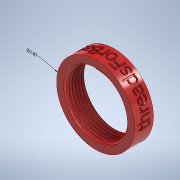
# Autodesk Inventor part: threadsForBaseV04
Saved by Autodesk Inventor 2021.1 (Build 251245010, 245A)
## iProperties
Created: 2020-08-18
Part Number: threadsForBaseV04
Material: PET Plastic
Document SubType Name: Modeling
Designer: robst
Density: 1.541 g/cm^3
Appearance: Red
Author: robst
Autodesk Inventor part; units mm, degrees
ref_plane "YZ Plane" through (0, 0, 0) normal (1, 0, 0) x (0, 1, 0)
ref_plane "XY Plane" through (0, 0, 0) normal (0, 0, 1) x (1, 0, 0)
sketch "Sketch3" plane through (0, 0, 0) normal (0, 0, 1) x (1, 0, 0)
  circle A0 centre (0, 0) radius 8.0645
  circle A1 centre (0, 0) radius 26.3436
  dimension "d8" = 16.129
  dimension "d9" = 52.6872
  constraints: 2 centre point, 2 coincident
  measures "d8" diameter of A0
  measures "d9" diameter of A1
extrude "Extrusion3" add sketch "Sketch3" along normal blind 44.45
sketch "Sketch4" plane through (0, 0, 44.45) normal (0, 0, 1) x (1, 0, 0)
  circle A0 centre (0, 0) radius 21.5811
  dimension "d12" = 43.1622
  constraints: 1 centre point, 1 coincident
  measures "d12" diameter of A0
extrude "Extrusion4" cut sketch "Sketch4" against normal blind 31.75
sketch "Sketch5" plane through (0, 0, 0) normal (1, 0, 0) x (0, 1, 0)
  line L0 (21.5811, 44.45) -> (21.5811, 12.7) projected
  line L1 (26.3436, 44.45) -> (-26.3436, 44.45) projected
  line L2 (21.5811, 44.45) -> (21.5811, 44.45)
  line L3 (21.5811, 44.45) -> (20.4572, 43.8011)
  line L4 (20.4572, 43.6031) -> (21.5811, 42.9542)
  arc A0 (20.4572, 43.8011) -> (20.4572, 43.6031) centre (20.5143, 43.7021) ccw
  line L5 (0, -8.89) -> (0, 53.34) construction
  line L6 (21.5811, 42.9542) -> (21.5811, 44.45)
  point P0 (0, 0)
  dimension "d15" = 60
  dimension "d17" = 0.1143
  dimension "d18" = 20.4
  dimension "d27" = 0
  constraints: 8 end point, 2 point on circle, 2 tangent, 1 centre point, 1 collinear, 1 equal length, 1 point on line, 1 vertical
  measures "d15" angle of L4 L3
  measures "d17" radius of A0
  measures "d18" distance edge to line of A0 L5
  measures "d27" distance of L2.end L0.start
coil "Coil2" sketch "Sketch5" operation add axis through (0, 0, -10) along (0, 0, -1) pitch 2.1167 turns 15 hand right
ref_plane "Work Plane3" through (0, 0, 31.75) normal (0, 0, 1) x (1, 0, 0)
sketch "Sketch12" plane through (0, 0, 31.75) normal (0, 0, 1) x (1, 0, 0)
  circle A0 centre (0, 0) radius 26.9875
  constraints: 1 centre point, 1 coincident
extrude "Extrusion7" cut sketch "Sketch12" against normal through all
ref_plane "Work Plane5" through (0, 26.3436, 0) normal (0, 1, 0) x (-1, 0, 0)
sketch "Sketch15" plane through (0, 26.3436, 0) normal (0, 1, 0) x (-1, 0, 0)
  line L0 (-26.3436, 31.75) -> (-26.3436, 44.45) projected
  line L1 (26.3436, 31.75) -> (26.3436, 44.45) projected
  line L2 (-26.3436, 38.1) -> (26.3436, 38.1) construction
  spline S0 degree 2 poles (-43.7594, 34.1788) (-44.5437, 34.1788) (-45.4267, 35.0742) (-45.4267, 36.0437) knots 0 0 0 1 2 2 2
  line L3 (-45.4267, 36.0437) -> (-45.4267, 39.2115)
  line L4 (-45.4267, 39.2115) -> (-46.0751, 39.2115)
  line L5 (-46.0751, 39.2115) -> (-46.0751, 40.0081)
  line L6 (-46.0751, 40.0081) -> (-45.4267, 40.0081)
  line L7 (-45.4267, 40.0081) -> (-45.4267, 41.6506)
  line L8 (-45.4267, 41.6506) -> (-44.4634, 41.6506)
  line L9 (-44.4634, 41.6506) -> (-44.4634, 40.0081)
  line L10 (-44.4634, 40.0081) -> (-42.6911, 40.0081)
  line L11 (-42.6911, 40.0081) -> (-42.6911, 39.2115)
  line L12 (-42.6911, 39.2115) -> (-44.4634, 39.2115)
  line L13 (-44.4634, 39.2115) -> (-44.4634, 36.4883)
  spline S1 degree 2 poles (-44.4634, 36.4883) (-44.4634, 36.0561) (-44.4325, 35.5806) (-44.3275, 35.3768) knots 0 0 0 1 2 2 2
  spline S2 degree 2 poles (-44.3275, 35.3768) (-44.2411, 35.1977) (-43.8521, 35.0187) (-43.5186, 35.0187) knots 0 0 0 1 2 2 2
  spline S3 degree 2 poles (-43.5186, 35.0187) (-43.2839, 35.0187) (-42.8455, 35.1607) (-42.7467, 35.2039) knots 0 0 0 1 2 2 2
  line L14 (-42.7467, 35.2039) -> (-42.6911, 35.2039)
  line L15 (-42.6911, 35.2039) -> (-42.6911, 34.3394)
  spline S4 degree 2 poles (-42.6911, 34.3394) (-42.9628, 34.2653) (-43.5186, 34.1788) (-43.7594, 34.1788) knots 0 0 0 1 2 2 2
  line L16 (-37.4918, 34.29) -> (-38.4551, 34.29)
  line L17 (-38.4551, 34.29) -> (-38.4551, 37.5504)
  spline S5 degree 2 poles (-38.4551, 37.5504) (-38.4551, 37.9456) (-38.5292, 38.6249) (-38.6403, 38.8287) knots 0 0 0 1 2 2 2
  spline S6 degree 2 poles (-38.6403, 38.8287) (-38.7576, 39.0448) (-39.1775, 39.2547) (-39.5357, 39.2547) knots 0 0 0 1 2 2 2
  spline S7 degree 2 poles (-39.5357, 39.2547) (-39.8939, 39.2547) (-40.6534, 38.8719) (-41.0177, 38.5631) knots 0 0 0 1 2 2 2
  line L18 (-41.0177, 38.5631) -> (-41.0177, 34.29)
  line L19 (-41.0177, 34.29) -> (-41.981, 34.29)
  line L20 (-41.981, 34.29) -> (-41.981, 42.2496)
  line L21 (-41.981, 42.2496) -> (-41.0177, 42.2496)
  line L22 (-41.0177, 42.2496) -> (-41.0177, 39.3721)
  spline S8 degree 2 poles (-41.0177, 39.3721) (-40.5855, 39.7611) (-39.7518, 40.1686) (-39.2825, 40.1686) knots 0 0 0 1 2 2 2
  spline S9 degree 2 poles (-39.2825, 40.1686) (-38.4427, 40.1686) (-37.4918, 39.0571) (-37.4918, 38.0012) knots 0 0 0 1 2 2 2
  line L23 (-37.4918, 38.0012) -> (-37.4918, 34.29)
  line L24 (-33.1075, 38.9769) -> (-33.1569, 38.9769)
  spline S10 degree 2 poles (-33.1569, 38.9769) (-33.268, 39.0077) (-33.5089, 39.0201) (-33.6756, 39.0201) knots 0 0 0 1 2 2 2
  spline S11 degree 2 poles (-33.6756, 39.0201) (-34.0646, 39.0201) (-34.8303, 38.6805) (-35.1761, 38.347) knots 0 0 0 1 2 2 2
  line L25 (-35.1761, 38.347) -> (-35.1761, 34.29)
  line L26 (-35.1761, 34.29) -> (-36.1394, 34.29)
  line L27 (-36.1394, 34.29) -> (-36.1394, 40.0081)
  line L28 (-36.1394, 40.0081) -> (-35.1761, 40.0081)
  line L29 (-35.1761, 40.0081) -> (-35.1761, 39.1559)
  spline S12 degree 2 poles (-35.1761, 39.1559) (-34.6512, 39.6252) (-33.867, 40.0081) (-33.4965, 40.0081) knots 0 0 0 1 2 2 2
  spline S13 degree 2 poles (-33.4965, 40.0081) (-33.3483, 40.0081) (-33.2001, 39.9957) (-33.1075, 39.9772) knots 0 0 0 1 2 2 2
  line L30 (-33.1075, 39.9772) -> (-33.1075, 38.9769)
  spline S14 degree 2 poles (-29.8779, 34.1603) (-31.2488, 34.1603) (-32.7555, 35.6979) (-32.7555, 37.1182) knots 0 0 0 1 2 2 2
  spline S15 degree 2 poles (-32.7555, 37.1182) (-32.7555, 38.5137) (-31.292, 40.1686) (-30.1126, 40.1686) knots 0 0 0 1 2 2 2
  spline S16 degree 2 poles (-30.1126, 40.1686) (-29.5815, 40.1686) (-28.7603, 39.8599) (-28.4577, 39.5326) knots 0 0 0 1 2 2 2
  spline S17 degree 2 poles (-28.4577, 39.5326) (-28.1489, 39.2053) (-27.8216, 38.2606) (-27.8216, 37.5751) knots 0 0 0 1 2 2 2
  line L31 (-27.8216, 37.5751) -> (-27.8216, 37.0502)
  line L32 (-27.8216, 37.0502) -> (-31.7798, 37.0502)
  spline S18 degree 2 poles (-31.7798, 37.0502) (-31.7798, 36.0561) (-30.7795, 35.0001) (-29.8903, 35.0001) knots 0 0 0 1 2 2 2
  spline S19 degree 2 poles (-29.8903, 35.0001) (-29.5754, 35.0001) (-28.964, 35.1422) (-28.717, 35.2533) knots 0 0 0 1 2 2 2
  spline S20 degree 2 poles (-28.717, 35.2533) (-28.4577, 35.3768) (-28.0995, 35.5929) (-27.9822, 35.6917) knots 0 0 0 1 2 2 2
  line L33 (-27.9822, 35.6917) -> (-27.9266, 35.6917)
  line L34 (-27.9266, 35.6917) -> (-27.9266, 34.642)
  spline S21 degree 2 poles (-27.9266, 34.642) (-28.0933, 34.5741) (-28.5997, 34.3765) (-28.7973, 34.3209) knots 0 0 0 1 2 2 2
  spline S22 degree 2 poles (-28.7973, 34.3209) (-29.0752, 34.2406) (-29.5321, 34.1603) (-29.8779, 34.1603) knots 0 0 0 1 2 2 2
  spline S23 degree 2 poles (-28.7603, 37.7851) (-28.7726, 38.1741) (-28.9332, 38.7422) (-29.0875, 38.9336) knots 0 0 0 1 2 2 2
  spline S24 degree 2 poles (-29.0875, 38.9336) (-29.2543, 39.1498) (-29.7791, 39.3782) (-30.1682, 39.3782) knots 0 0 0 1 2 2 2
  spline S25 degree 2 poles (-30.1682, 39.3782) (-30.551, 39.3782) (-31.0882, 39.1498) (-31.3105, 38.9275) knots 0 0 0 1 2 2 2
  spline S26 degree 2 poles (-31.3105, 38.9275) (-31.5267, 38.699) (-31.749, 38.1494) (-31.7798, 37.7851) knots 0 0 0 1 2 2 2
  line L35 (-31.7798, 37.7851) -> (-28.7603, 37.7851)
  spline S27 degree 2 poles (-23.6597, 34.8952) (-23.777, 34.8087) (-24.1722, 34.5) (-24.3574, 34.4073) knots 0 0 0 1 2 2 2
  spline S28 degree 2 poles (-24.3574, 34.4073) (-24.6106, 34.2715) (-25.0861, 34.1294) (-25.5184, 34.1294) knots 0 0 0 1 2 2 2
  spline S29 degree 2 poles (-25.5184, 34.1294) (-25.8703, 34.1294) (-26.5064, 34.395) (-26.7472, 34.6358) knots 0 0 0 1 2 2 2
  spline S30 degree 2 poles (-26.7472, 34.6358) (-26.9757, 34.8705) (-27.2535, 35.5621) (-27.2535, 35.9449) knots 0 0 0 1 2 2 2
  spline S31 degree 2 poles (-27.2535, 35.9449) (-27.2535, 36.5377) (-26.7534, 37.3775) (-26.21, 37.6183) knots 0 0 0 1 2 2 2
  spline S32 degree 2 poles (-26.21, 37.6183) (-25.7283, 37.8406) (-24.4192, 38.0074) (-23.6597, 38.0506) knots 0 0 0 1 2 2 2
  line L36 (-23.6597, 38.0506) -> (-23.6597, 38.2359)
  spline S33 degree 2 poles (-23.6597, 38.2359) (-23.6597, 38.5693) (-23.8634, 38.983) (-24.0487, 39.1004) knots 0 0 0 1 2 2 2
  spline S34 degree 2 poles (-24.0487, 39.1004) (-24.2339, 39.2177) (-24.765, 39.2918) (-25.0491, 39.2918) knots 0 0 0 1 2 2 2
  spline S35 degree 2 poles (-25.0491, 39.2918) (-25.3825, 39.2918) (-26.2841, 39.0942) (-26.7348, 38.9028) knots 0 0 0 1 2 2 2
  line L37 (-26.7348, 38.9028) -> (-26.7904, 38.9028)
  line L38 (-26.7904, 38.9028) -> (-26.7904, 39.8846)
  spline S36 degree 2 poles (-26.7904, 39.8846) (-26.5249, 39.9587) (-25.5307, 40.1439) (-25.0429, 40.1439) knots 0 0 0 1 2 2 2
  spline S37 degree 2 poles (-25.0429, 40.1439) (-24.4501, 40.1439) (-23.6411, 39.9587) (-23.32, 39.7179) knots 0 0 0 1 2 2 2
  spline S38 degree 2 poles (-23.32, 39.7179) (-23.0051, 39.4832) (-22.6964, 38.736) (-22.6964, 38.1988) knots 0 0 0 1 2 2 2
  line L39 (-22.6964, 38.1988) -> (-22.6964, 34.29)
  line L40 (-22.6964, 34.29) -> (-23.6597, 34.29)
  line L41 (-23.6597, 34.29) -> (-23.6597, 34.8952)
  line L42 (-23.6597, 35.6979) -> (-23.6597, 37.2849)
  spline S39 degree 2 poles (-23.6597, 37.2849) (-24.0055, 37.254) (-25.0491, 37.149) (-25.3763, 37.0502) knots 0 0 0 1 2 2 2
  spline S40 degree 2 poles (-25.3763, 37.0502) (-25.7592, 36.9329) (-26.2594, 36.4451) (-26.2594, 36.0128) knots 0 0 0 1 2 2 2
  spline S41 degree 2 poles (-26.2594, 36.0128) (-26.2594, 35.5188) (-25.7036, 35.0187) (-25.1726, 35.0187) knots 0 0 0 1 2 2 2
  spline S42 degree 2 poles (-25.1726, 35.0187) (-24.7218, 35.0187) (-23.9808, 35.4077) (-23.6597, 35.6979) knots 0 0 0 1 2 2 2
  line L43 (-16.9474, 34.29) -> (-17.9107, 34.29)
  line L44 (-17.9107, 34.29) -> (-17.9107, 34.8705)
  spline S43 degree 2 poles (-17.9107, 34.8705) (-18.133, 34.6852) (-18.4603, 34.4382) (-18.6826, 34.3332) knots 0 0 0 1 2 2 2
  spline S44 degree 2 poles (-18.6826, 34.3332) (-18.8864, 34.2344) (-19.3248, 34.1294) (-19.615, 34.1294) knots 0 0 0 1 2 2 2
  spline S45 degree 2 poles (-19.615, 34.1294) (-20.0843, 34.1294) (-20.8747, 34.5185) (-21.1526, 34.8952) knots 0 0 0 1 2 2 2
  spline S46 degree 2 poles (-21.1526, 34.8952) (-21.4305, 35.2718) (-21.7392, 36.3833) (-21.7392, 37.1058) knots 0 0 0 1 2 2 2
  spline S47 degree 2 poles (-21.7392, 37.1058) (-21.7392, 37.8592) (-21.3502, 38.9583) (-21.0106, 39.3721) knots 0 0 0 1 2 2 2
  spline S48 degree 2 poles (-21.0106, 39.3721) (-20.6957, 39.7426) (-19.8126, 40.1686) (-19.3248, 40.1686) knots 0 0 0 1 2 2 2
  spline S49 degree 2 poles (-19.3248, 40.1686) (-18.8987, 40.1686) (-18.2627, 39.9772) (-17.9107, 39.7796) knots 0 0 0 1 2 2 2
  line L45 (-17.9107, 39.7796) -> (-17.9107, 42.2496)
  line L46 (-17.9107, 42.2496) -> (-16.9474, 42.2496)
  line L47 (-16.9474, 42.2496) -> (-16.9474, 34.29)
  line L48 (-17.9107, 35.6794) -> (-17.9107, 38.983)
  spline S50 degree 2 poles (-17.9107, 38.983) (-18.2689, 39.1559) (-18.837, 39.2856) (-19.1642, 39.2856) knots 0 0 0 1 2 2 2
  spline S51 degree 2 poles (-19.1642, 39.2856) (-19.9052, 39.2856) (-20.7451, 38.1741) (-20.7451, 37.1243) knots 0 0 0 1 2 2 2
  spline S52 degree 2 poles (-20.7451, 37.1243) (-20.7451, 36.1116) (-20.1028, 35.0434) (-19.3927, 35.0434) knots 0 0 0 1 2 2 2
  spline S53 degree 2 poles (-19.3927, 35.0434) (-19.016, 35.0434) (-18.2503, 35.3892) (-17.9107, 35.6794) knots 0 0 0 1 2 2 2
  spline S54 degree 2 poles (-14.0081, 34.1541) (-14.5824, 34.1541) (-15.5765, 34.4629) (-15.9038, 34.6358) knots 0 0 0 1 2 2 2
  line L49 (-15.9038, 34.6358) -> (-15.9038, 35.7164)
  line L50 (-15.9038, 35.7164) -> (-15.8544, 35.7164)
  spline S55 degree 2 poles (-15.8544, 35.7164) (-15.7309, 35.6176) (-15.3975, 35.383) (-15.1196, 35.2533) knots 0 0 0 1 2 2 2
  spline S56 degree 2 poles (-15.1196, 35.2533) (-14.8788, 35.136) (-14.286, 34.9631) (-13.971, 34.9631) knots 0 0 0 1 2 2 2
  spline S57 degree 2 poles (-13.971, 34.9631) (-13.7426, 34.9631) (-13.2177, 35.0681) (-13.0942, 35.1545) knots 0 0 0 1 2 2 2
  spline S58 degree 2 poles (-13.0942, 35.1545) (-12.9151, 35.2718) (-12.7545, 35.5374) (-12.7545, 35.8091) knots 0 0 0 1 2 2 2
  spline S59 degree 2 poles (-12.7545, 35.8091) (-12.7545, 36.1487) (-13.1251, 36.5007) (-13.6005, 36.618) knots 0 0 0 1 2 2 2
  spline S60 degree 2 poles (-13.6005, 36.618) (-13.7858, 36.6612) (-14.3786, 36.7847) (-14.6318, 36.8526) knots 0 0 0 1 2 2 2
  spline S61 degree 2 poles (-14.6318, 36.8526) (-15.2863, 37.0441) (-15.8791, 37.8345) (-15.8791, 38.3964) knots 0 0 0 1 2 2 2
  spline S62 degree 2 poles (-15.8791, 38.3964) (-15.8791, 39.1745) (-14.712, 40.1439) (-13.7487, 40.1439) knots 0 0 0 1 2 2 2
  spline S63 degree 2 poles (-13.7487, 40.1439) (-13.2733, 40.1439) (-12.3099, 39.9093) (-11.9827, 39.7302) knots 0 0 0 1 2 2 2
  line L51 (-11.9827, 39.7302) -> (-11.9827, 38.699)
  line L52 (-11.9827, 38.699) -> (-12.0321, 38.699)
  spline S64 degree 2 poles (-12.0321, 38.699) (-12.4026, 38.9954) (-13.3041, 39.335) (-13.7673, 39.335) knots 0 0 0 1 2 2 2
  spline S65 degree 2 poles (-13.7673, 39.335) (-14.2427, 39.335) (-14.8973, 38.9336) (-14.8973, 38.5323) knots 0 0 0 1 2 2 2
  spline S66 degree 2 poles (-14.8973, 38.5323) (-14.8973, 38.1679) (-14.5083, 37.8159) (-14.076, 37.7048) knots 0 0 0 1 2 2 2
  spline S67 degree 2 poles (-14.076, 37.7048) (-13.8661, 37.6492) (-13.335, 37.5381) (-13.0448, 37.4701) knots 0 0 0 1 2 2 2
  spline S68 degree 2 poles (-13.0448, 37.4701) (-12.4149, 37.3096) (-11.7727, 36.5748) (-11.7727, 35.9387) knots 0 0 0 1 2 2 2
  spline S69 degree 2 poles (-11.7727, 35.9387) (-11.7727, 35.5682) (-12.0629, 34.9137) (-12.347, 34.6729) knots 0 0 0 1 2 2 2
  spline S70 degree 2 poles (-12.347, 34.6729) (-12.6496, 34.4197) (-13.4215, 34.1541) (-14.0081, 34.1541) knots 0 0 0 1 2 2 2
  line L53 (-6.2461, 41.0084) -> (-9.7905, 41.0084)
  line L54 (-9.7905, 41.0084) -> (-9.7905, 38.8595)
  line L55 (-9.7905, 38.8595) -> (-6.3943, 38.8595)
  line L56 (-6.3943, 38.8595) -> (-6.3943, 37.958)
  line L57 (-6.3943, 37.958) -> (-9.7905, 37.958)
  line L58 (-9.7905, 37.958) -> (-9.7905, 34.29)
  line L59 (-9.7905, 34.29) -> (-10.8032, 34.29)
  line L60 (-10.8032, 34.29) -> (-10.8032, 41.91)
  line L61 (-10.8032, 41.91) -> (-6.2461, 41.91)
  line L62 (-6.2461, 41.91) -> (-6.2461, 41.0084)
  spline S71 degree 2 poles (-0.7132, 37.149) (-0.7132, 35.7041) (-2.1026, 34.1294) (-3.2635, 34.1294) knots 0 0 0 1 2 2 2
  spline S72 degree 2 poles (-3.2635, 34.1294) (-4.4553, 34.1294) (-5.82, 35.7535) (-5.82, 37.149) knots 0 0 0 1 2 2 2
  spline S73 degree 2 poles (-5.82, 37.149) (-5.82, 38.5817) (-4.4121, 40.1686) (-3.2635, 40.1686) knots 0 0 0 1 2 2 2
  spline S74 degree 2 poles (-3.2635, 40.1686) (-2.1026, 40.1686) (-0.7132, 38.5878) (-0.7132, 37.149) knots 0 0 0 1 2 2 2
  spline S75 degree 2 poles (-1.7074, 37.149) (-1.7074, 38.2606) (-2.5163, 39.3412) (-3.2635, 39.3412) knots 0 0 0 1 2 2 2
  spline S76 degree 2 poles (-3.2635, 39.3412) (-4.0107, 39.3412) (-4.8258, 38.2606) (-4.8258, 37.149) knots 0 0 0 1 2 2 2
  spline S77 degree 2 poles (-4.8258, 37.149) (-4.8258, 36.0684) (-4.0107, 34.9569) (-3.2635, 34.9569) knots 0 0 0 1 2 2 2
  spline S78 degree 2 poles (-3.2635, 34.9569) (-2.5225, 34.9569) (-1.7074, 36.0499) (-1.7074, 37.149) knots 0 0 0 1 2 2 2
  line L63 (3.3067, 38.9769) -> (3.2573, 38.9769)
  spline S79 degree 2 poles (3.2573, 38.9769) (3.1462, 39.0077) (2.9054, 39.0201) (2.7386, 39.0201) knots 0 0 0 1 2 2 2
  spline S80 degree 2 poles (2.7386, 39.0201) (2.3496, 39.0201) (1.5839, 38.6805) (1.2381, 38.347) knots 0 0 0 1 2 2 2
  line L64 (1.2381, 38.347) -> (1.2381, 34.29)
  line L65 (1.2381, 34.29) -> (0.2748, 34.29)
  line L66 (0.2748, 34.29) -> (0.2748, 40.0081)
  line L67 (0.2748, 40.0081) -> (1.2381, 40.0081)
  line L68 (1.2381, 40.0081) -> (1.2381, 39.1559)
  spline S81 degree 2 poles (1.2381, 39.1559) (1.763, 39.6252) (2.5472, 40.0081) (2.9177, 40.0081) knots 0 0 0 1 2 2 2
  spline S82 degree 2 poles (2.9177, 40.0081) (3.0659, 40.0081) (3.2141, 39.9957) (3.3067, 39.9772) knots 0 0 0 1 2 2 2
  line L69 (3.3067, 39.9772) -> (3.3067, 38.9769)
  spline S83 degree 2 poles (9.2965, 36.6303) (9.2965, 36.0622) (8.8643, 35.1916) (8.5061, 34.9075) knots 0 0 0 1 2 2 2
  spline S84 degree 2 poles (8.5061, 34.9075) (8.0739, 34.5741) (7.092, 34.29) (6.314, 34.29) knots 0 0 0 1 2 2 2
  line L70 (6.314, 34.29) -> (4.128, 34.29)
  line L71 (4.128, 34.29) -> (4.128, 41.91)
  line L72 (4.128, 41.91) -> (6.1473, 41.91)
  spline S85 degree 2 poles (6.1473, 41.91) (6.9624, 41.91) (7.7775, 41.805) (8.148, 41.6012) knots 0 0 0 1 2 2 2
  spline S86 degree 2 poles (8.148, 41.6012) (8.5617, 41.3851) (8.9384, 40.675) (8.9384, 40.1933) knots 0 0 0 1 2 2 2
  spline S87 degree 2 poles (8.9384, 40.1933) (8.9384, 39.6561) (8.3703, 38.804) (7.8701, 38.5631) knots 0 0 0 1 2 2 2
  line L73 (7.8701, 38.5631) -> (7.8701, 38.5261)
  spline S88 degree 2 poles (7.8701, 38.5261) (8.5493, 38.3408) (9.2965, 37.359) (9.2965, 36.6303) knots 0 0 0 1 2 2 2
  spline S89 degree 2 poles (8.2406, 36.5871) (8.2406, 37.0194) (7.9936, 37.5751) (7.6231, 37.7727) knots 0 0 0 1 2 2 2
  spline S90 degree 2 poles (7.6231, 37.7727) (7.3823, 37.8962) (6.8142, 37.9703) (6.2893, 37.9703) knots 0 0 0 1 2 2 2
  line L74 (6.2893, 37.9703) -> (5.1407, 37.9703)
  line L75 (5.1407, 37.9703) -> (5.1407, 35.1545)
  line L76 (5.1407, 35.1545) -> (5.962, 35.1545)
  spline S91 degree 2 poles (5.962, 35.1545) (6.6289, 35.1545) (7.3946, 35.278) (7.691, 35.4756) knots 0 0 0 1 2 2 2
  spline S92 degree 2 poles (7.691, 35.4756) (7.9751, 35.6794) (8.2406, 36.1857) (8.2406, 36.5871) knots 0 0 0 1 2 2 2
  spline S93 degree 2 poles (7.8824, 40.0513) (7.8824, 40.323) (7.6972, 40.7306) (7.4934, 40.8479) knots 0 0 0 1 2 2 2
  spline S94 degree 2 poles (7.4934, 40.8479) (7.2464, 40.9837) (6.6474, 41.0455) (6.1102, 41.0455) knots 0 0 0 1 2 2 2
  line L77 (6.1102, 41.0455) -> (5.1407, 41.0455)
  line L78 (5.1407, 41.0455) -> (5.1407, 38.8163)
  line L79 (5.1407, 38.8163) -> (6.2893, 38.8163)
  spline S95 degree 2 poles (6.2893, 38.8163) (6.7648, 38.8163) (7.2155, 38.9151) (7.4564, 39.0695) knots 0 0 0 1 2 2 2
  spline S96 degree 2 poles (7.4564, 39.0695) (7.691, 39.2177) (7.8824, 39.6932) (7.8824, 40.0513) knots 0 0 0 1 2 2 2
  spline S97 degree 2 poles (13.4153, 34.8952) (13.2979, 34.8087) (12.9027, 34.5) (12.7175, 34.4073) knots 0 0 0 1 2 2 2
  spline S98 degree 2 poles (12.7175, 34.4073) (12.4643, 34.2715) (11.9888, 34.1294) (11.5566, 34.1294) knots 0 0 0 1 2 2 2
  spline S99 degree 2 poles (11.5566, 34.1294) (11.2046, 34.1294) (10.5686, 34.395) (10.3278, 34.6358) knots 0 0 0 1 2 2 2
  spline S100 degree 2 poles (10.3278, 34.6358) (10.0993, 34.8705) (9.8214, 35.5621) (9.8214, 35.9449) knots 0 0 0 1 2 2 2
  spline S101 degree 2 poles (9.8214, 35.9449) (9.8214, 36.5377) (10.3216, 37.3775) (10.865, 37.6183) knots 0 0 0 1 2 2 2
  spline S102 degree 2 poles (10.865, 37.6183) (11.3466, 37.8406) (12.6557, 38.0074) (13.4153, 38.0506) knots 0 0 0 1 2 2 2
  line L80 (13.4153, 38.0506) -> (13.4153, 38.2359)
  spline S103 degree 2 poles (13.4153, 38.2359) (13.4153, 38.5693) (13.2115, 38.983) (13.0262, 39.1004) knots 0 0 0 1 2 2 2
  spline S104 degree 2 poles (13.0262, 39.1004) (12.841, 39.2177) (12.3099, 39.2918) (12.0259, 39.2918) knots 0 0 0 1 2 2 2
  spline S105 degree 2 poles (12.0259, 39.2918) (11.6924, 39.2918) (10.7909, 39.0942) (10.3401, 38.9028) knots 0 0 0 1 2 2 2
  line L81 (10.3401, 38.9028) -> (10.2845, 38.9028)
  line L82 (10.2845, 38.9028) -> (10.2845, 39.8846)
  spline S106 degree 2 poles (10.2845, 39.8846) (10.5501, 39.9587) (11.5442, 40.1439) (12.0321, 40.1439) knots 0 0 0 1 2 2 2
  spline S107 degree 2 poles (12.0321, 40.1439) (12.6249, 40.1439) (13.4338, 39.9587) (13.7549, 39.7179) knots 0 0 0 1 2 2 2
  spline S108 degree 2 poles (13.7549, 39.7179) (14.0698, 39.4832) (14.3786, 38.736) (14.3786, 38.1988) knots 0 0 0 1 2 2 2
  line L83 (14.3786, 38.1988) -> (14.3786, 34.29)
  line L84 (14.3786, 34.29) -> (13.4153, 34.29)
  line L85 (13.4153, 34.29) -> (13.4153, 34.8952)
  line L86 (13.4153, 35.6979) -> (13.4153, 37.2849)
  spline S109 degree 2 poles (13.4153, 37.2849) (13.0695, 37.254) (12.0259, 37.149) (11.6986, 37.0502) knots 0 0 0 1 2 2 2
  spline S110 degree 2 poles (11.6986, 37.0502) (11.3158, 36.9329) (10.8156, 36.4451) (10.8156, 36.0128) knots 0 0 0 1 2 2 2
  spline S111 degree 2 poles (10.8156, 36.0128) (10.8156, 35.5188) (11.3713, 35.0187) (11.9024, 35.0187) knots 0 0 0 1 2 2 2
  spline S112 degree 2 poles (11.9024, 35.0187) (12.3532, 35.0187) (13.0942, 35.4077) (13.4153, 35.6979) knots 0 0 0 1 2 2 2
  spline S113 degree 2 poles (17.2747, 34.1541) (16.7004, 34.1541) (15.7062, 34.4629) (15.3789, 34.6358) knots 0 0 0 1 2 2 2
  line L87 (15.3789, 34.6358) -> (15.3789, 35.7164)
  line L88 (15.3789, 35.7164) -> (15.4283, 35.7164)
  spline S114 degree 2 poles (15.4283, 35.7164) (15.5518, 35.6176) (15.8853, 35.383) (16.1632, 35.2533) knots 0 0 0 1 2 2 2
  spline S115 degree 2 poles (16.1632, 35.2533) (16.404, 35.136) (16.9968, 34.9631) (17.3117, 34.9631) knots 0 0 0 1 2 2 2
  spline S116 degree 2 poles (17.3117, 34.9631) (17.5402, 34.9631) (18.0651, 35.0681) (18.1886, 35.1545) knots 0 0 0 1 2 2 2
  spline S117 degree 2 poles (18.1886, 35.1545) (18.3677, 35.2718) (18.5282, 35.5374) (18.5282, 35.8091) knots 0 0 0 1 2 2 2
  spline S118 degree 2 poles (18.5282, 35.8091) (18.5282, 36.1487) (18.1577, 36.5007) (17.6822, 36.618) knots 0 0 0 1 2 2 2
  spline S119 degree 2 poles (17.6822, 36.618) (17.497, 36.6612) (16.9042, 36.7847) (16.651, 36.8526) knots 0 0 0 1 2 2 2
  spline S120 degree 2 poles (16.651, 36.8526) (15.9964, 37.0441) (15.4036, 37.8345) (15.4036, 38.3964) knots 0 0 0 1 2 2 2
  spline S121 degree 2 poles (15.4036, 38.3964) (15.4036, 39.1745) (16.5707, 40.1439) (17.534, 40.1439) knots 0 0 0 1 2 2 2
  spline S122 degree 2 poles (17.534, 40.1439) (18.0095, 40.1439) (18.9728, 39.9093) (19.3001, 39.7302) knots 0 0 0 1 2 2 2
  line L89 (19.3001, 39.7302) -> (19.3001, 38.699)
  line L90 (19.3001, 38.699) -> (19.2507, 38.699)
  spline S123 degree 2 poles (19.2507, 38.699) (18.8802, 38.9954) (17.9786, 39.335) (17.5155, 39.335) knots 0 0 0 1 2 2 2
  spline S124 degree 2 poles (17.5155, 39.335) (17.04, 39.335) (16.3855, 38.9336) (16.3855, 38.5323) knots 0 0 0 1 2 2 2
  spline S125 degree 2 poles (16.3855, 38.5323) (16.3855, 38.1679) (16.7745, 37.8159) (17.2067, 37.7048) knots 0 0 0 1 2 2 2
  spline S126 degree 2 poles (17.2067, 37.7048) (17.4167, 37.6492) (17.9478, 37.5381) (18.238, 37.4701) knots 0 0 0 1 2 2 2
  spline S127 degree 2 poles (18.238, 37.4701) (18.8678, 37.3096) (19.51, 36.5748) (19.51, 35.9387) knots 0 0 0 1 2 2 2
  spline S128 degree 2 poles (19.51, 35.9387) (19.51, 35.5682) (19.2198, 34.9137) (18.9358, 34.6729) knots 0 0 0 1 2 2 2
  spline S129 degree 2 poles (18.9358, 34.6729) (18.6332, 34.4197) (17.8613, 34.1541) (17.2747, 34.1541) knots 0 0 0 1 2 2 2
  spline S130 degree 2 poles (22.8878, 34.1603) (21.5169, 34.1603) (20.0102, 35.6979) (20.0102, 37.1182) knots 0 0 0 1 2 2 2
  spline S131 degree 2 poles (20.0102, 37.1182) (20.0102, 38.5137) (21.4737, 40.1686) (22.6531, 40.1686) knots 0 0 0 1 2 2 2
  spline S132 degree 2 poles (22.6531, 40.1686) (23.1842, 40.1686) (24.0055, 39.8599) (24.308, 39.5326) knots 0 0 0 1 2 2 2
  spline S133 degree 2 poles (24.308, 39.5326) (24.6168, 39.2053) (24.9441, 38.2606) (24.9441, 37.5751) knots 0 0 0 1 2 2 2
  line L91 (24.9441, 37.5751) -> (24.9441, 37.0502)
  line L92 (24.9441, 37.0502) -> (20.9859, 37.0502)
  spline S134 degree 2 poles (20.9859, 37.0502) (20.9859, 36.0561) (21.9862, 35.0001) (22.8754, 35.0001) knots 0 0 0 1 2 2 2
  spline S135 degree 2 poles (22.8754, 35.0001) (23.1904, 35.0001) (23.8017, 35.1422) (24.0487, 35.2533) knots 0 0 0 1 2 2 2
  spline S136 degree 2 poles (24.0487, 35.2533) (24.308, 35.3768) (24.6662, 35.5929) (24.7835, 35.6917) knots 0 0 0 1 2 2 2
  line L93 (24.7835, 35.6917) -> (24.8391, 35.6917)
  line L94 (24.8391, 35.6917) -> (24.8391, 34.642)
  spline S137 degree 2 poles (24.8391, 34.642) (24.6724, 34.5741) (24.166, 34.3765) (23.9684, 34.3209) knots 0 0 0 1 2 2 2
  spline S138 degree 2 poles (23.9684, 34.3209) (23.6905, 34.2406) (23.2336, 34.1603) (22.8878, 34.1603) knots 0 0 0 1 2 2 2
  spline S139 degree 2 poles (24.0055, 37.7851) (23.9931, 38.1741) (23.8326, 38.7422) (23.6782, 38.9336) knots 0 0 0 1 2 2 2
  spline S140 degree 2 poles (23.6782, 38.9336) (23.5115, 39.1498) (22.9866, 39.3782) (22.5976, 39.3782) knots 0 0 0 1 2 2 2
  spline S141 degree 2 poles (22.5976, 39.3782) (22.2147, 39.3782) (21.6775, 39.1498) (21.4552, 38.9275) knots 0 0 0 1 2 2 2
  spline S142 degree 2 poles (21.4552, 38.9275) (21.2391, 38.699) (21.0167, 38.1494) (20.9859, 37.7851) knots 0 0 0 1 2 2 2
  line L95 (20.9859, 37.7851) -> (24.0055, 37.7851)
  line L96 (34.7933, 41.91) -> (32.1689, 34.29)
  line L97 (32.1689, 34.29) -> (31.0759, 34.29)
  line L98 (31.0759, 34.29) -> (28.4515, 41.91)
  line L99 (28.4515, 41.91) -> (29.5383, 41.91)
  line L100 (29.5383, 41.91) -> (31.6502, 35.5806)
  line L101 (31.6502, 35.5806) -> (33.762, 41.91)
  line L102 (33.762, 41.91) -> (34.7933, 41.91)
  spline S143 degree 2 poles (40.1347, 38.1) (40.1347, 36.0499) (38.9429, 34.1294) (37.7017, 34.1294) knots 0 0 0 1 2 2 2
  spline S144 degree 2 poles (37.7017, 34.1294) (36.442, 34.1294) (35.2626, 36.0869) (35.2626, 38.0938) knots 0 0 0 1 2 2 2
  spline S145 degree 2 poles (35.2626, 38.0938) (35.2626, 40.1563) (36.4544, 42.0644) (37.7017, 42.0644) knots 0 0 0 1 2 2 2
  spline S146 degree 2 poles (37.7017, 42.0644) (38.9552, 42.0644) (40.1347, 40.0884) (40.1347, 38.1) knots 0 0 0 1 2 2 2
  spline S147 degree 2 poles (38.8256, 35.7782) (38.9738, 36.1549) (39.0973, 37.3158) (39.0973, 38.1) knots 0 0 0 1 2 2 2
  spline S148 degree 2 poles (39.0973, 38.1) (39.0973, 38.8842) (38.9738, 40.039) (38.8194, 40.428) knots 0 0 0 1 2 2 2
  spline S149 degree 2 poles (38.8194, 40.428) (38.665, 40.817) (38.1278, 41.2184) (37.7017, 41.2184) knots 0 0 0 1 2 2 2
  spline S150 degree 2 poles (37.7017, 41.2184) (37.2756, 41.2184) (36.7261, 40.817) (36.5655, 40.4156) knots 0 0 0 1 2 2 2
  spline S151 degree 2 poles (36.5655, 40.4156) (36.4111, 40.0266) (36.3, 38.841) (36.3, 38.0938) knots 0 0 0 1 2 2 2
  spline S152 degree 2 poles (36.3, 38.0938) (36.3, 37.2911) (36.3988, 36.2166) (36.5593, 35.7967) knots 0 0 0 1 2 2 2
  spline S153 degree 2 poles (36.5593, 35.7967) (36.7075, 35.4015) (37.2571, 34.9754) (37.7017, 34.9754) knots 0 0 0 1 2 2 2
  spline S154 degree 2 poles (37.7017, 34.9754) (38.1216, 34.9754) (38.6712, 35.3768) (38.8256, 35.7782) knots 0 0 0 1 2 2 2
  line L103 (46.0133, 36.9082) -> (45.1056, 36.9082)
  line L104 (45.1056, 36.9082) -> (45.1056, 34.29)
  line L105 (45.1056, 34.29) -> (44.1238, 34.29)
  line L106 (44.1238, 34.29) -> (44.1238, 36.9082)
  line L107 (44.1238, 36.9082) -> (40.7584, 36.9082)
  line L108 (40.7584, 36.9082) -> (40.7584, 37.9827)
  line L109 (40.7584, 37.9827) -> (44.167, 41.91)
  line L110 (44.167, 41.91) -> (45.1056, 41.91)
  line L111 (45.1056, 41.91) -> (45.1056, 37.7295)
  line L112 (45.1056, 37.7295) -> (46.0133, 37.7295)
  line L113 (46.0133, 37.7295) -> (46.0133, 36.9082)
  line L114 (44.1238, 37.7295) -> (44.1238, 40.7059)
  line L115 (44.1238, 40.7059) -> (41.5611, 37.7295)
  line L116 (41.5611, 37.7295) -> (44.1238, 37.7295)
  point P0 (0, 0)
  constraints: 2 end point, 2 midpoint, 1 horizontal
emboss "Emboss2" sketch "Sketch15" operation cut depth 1.27 direction (0, -1, 0) wrap yes faces at (26.0025, 4.2258, 35.9833) contours S29 S30 S31 L0 | L0 S31 S32 L36 S33 S34 S35 S36 S37 S38 L39 L40 L41 S27 S28 S29 | S35 L37 L38 S36 L0 | S0 L3 L4 L5 L6 L7 L8 L9 L10 L11 L12 L13 S1 S2 S3 L14 L15 S4 | L16 L17 S5 S6 S7 L18 L19 L20 L21 L22 S8 S9 L23 | L24 S10 S11 L25 L26 L27 L28 L29 S12 S13 L30 | S14 S15 S16 S17 L31 L32 S18 S19 S20 L33 L34 S21 S22 | L43 L44 S43 S44 S45 S46 S47 S48 S49 L45 L46 L47 | S54 L49 L50 S55 S56 S57 S58 S59 S60 S61 S62 S63 L51 L52 S64 S65 S66 S67 S68 S69 S70 | L53 L54 L55 L56 L57 L58 L59 L60 L61 L62 | S71 S72 S73 S74 | L63 S79 S80 L64 L65 L66 L67 L68 S81 S82 L69 | S83 S84 L70 L71 L72 S85 S86 S87 L73 S88 | S97 S98 S99 S100 S101 S102 L80 S103 S104 S105 L81 L82 S106 S107 S108 L83 L84 L85 | S113 L87 L88 S114 S115 S116 S117 S118 S119 S120 S121 S122 L89 L90 S123 S124 S125 S126 S127 S128 S129 | S130 S131 S132 S133 L91 L92 S134 S135 S136 L93 L94 S137 S138 | L96 L97 L98 L99 L100 L101 L102 | S143 S144 S145 S146 | L103 L104 L105 L106 L107 L108 L109 L110 L111 L112 L113
equation "\"d8\" = innerDiameter"
equation "\"d9\" = outsideDiameter"
equation "\"d10\" = lengthOfBrakeStop"
equation "\"d12\" = b1MajorDiameterAvg"
equation "\"d13\" = depthOfThread"
equation "\"d17\" = b1RootRadiusAvg"
equation "\"d18\" = 0.5 * b1MinorDiameterAvg"
equation "\"d28\" = pitch"
equation "\"d29\" = depthOfThread"
equation "\"innerDiameter\" = 16.129"
equation "\"heightOfBrake\" = 6.35"
equation "\"majorDiameter\" = 41.22928"
equation "\"pitchDiameter\" = 39.85514"
equation "\"minorDiameter\" = 38.7096"
equation "\"crestFlat\" = 0.4318"
equation "\"rootRadius\" = 0.22352"
equation "\"threadDepth\" = 1.52146"
equation "\"outsideDiameter\" = 52.68722"
equation "\"lengthOfBrakeStop\" = 44.45"
equation "\"depthOfThread\" = lengthOfBrakeStop - brakeStopLength"
equation "\"brakeStopLength\" = 12.7"
equation "\"b1MajorDiameterAvg\" = 43.16222"
equation "\"b1MinorDiameterAvg\" = 40.80002"
equation "\"b1RootRadiusAvg\" = 0.1143"
equation "\"outsideRadius\" = 0.5 * outsideDiameter"
equation "\"d62\" = outsideRadius"
equation "\"pitch\" = 2.116667"
body "Solid2"
